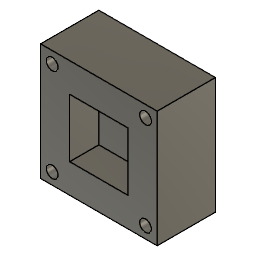
Milling (Autodesk Fusion 360 design; units mm, degrees)
part number: 2026-06-28-19-41-07-142
Autodesk Fusion 360 part; units mm, degrees
sketch "Sketch5" plane through (0, 0, 0) normal (0, 1, 0) x (1, 0, 0)
  line L0 (0, 0) -> (100, 0)
  line L1 (100, 0) -> (100, -100)
  line L2 (100, -100) -> (0, -100)
  line L3 (0, -100) -> (0, 0)
  line L4 (25, -75) -> (75, -75)
  line L5 (75, -75) -> (75, -25)
  line L6 (75, -25) -> (25, -25)
  line L7 (25, -25) -> (25, -75)
  circle A0 centre (10, -90) radius 5
  circle A1 centre (90, -90) radius 5
  circle A2 centre (90, -10) radius 5
  circle A3 centre (10, -10) radius 5
  dimension "d57" = 100
  dimension "d58" = 100
  dimension "d59" = 50
  dimension "d60" = 50
  dimension "d61" = 25
  dimension "d62" = 25
  dimension "d63" = 10
  dimension "d64" = 10
  dimension "d65" = 10
  dimension "d66" = 10
  constraint horizontal L0
  constraint vertical L1
  constraint horizontal L2
  constraint vertical L3
  constraint coincident L0.start L3.end
  constraint horizontal L4
  constraint vertical L5
  constraint horizontal L6
  constraint vertical L7
  measures "d57" distance of L1.end L2.end
  measures "d58" distance of L0.end L1.end
  measures "d59" distance of L4.start L4.end
  measures "d60" distance of L4.end L5.end
  measures "d61" distance of L1 L5
  measures "d62" distance of L2 L4
  measures "d63" diameter of A0
  measures "d64" diameter of A1
  measures "d65" diameter of A2
  measures "d66" diameter of A3
sketch "Sketch6" plane through (0, 0, 0) normal (0, 1, 0) x (1, 0, 0)
  line L0 (0, 0) -> (100, 0)
  line L1 (100, 0) -> (100, -100)
  line L2 (100, -100) -> (0, -100)
  line L3 (0, -100) -> (0, 0)
  line L4 (25, -75) -> (75, -75)
  line L5 (75, -75) -> (75, -25)
  line L6 (75, -25) -> (25, -25)
  line L7 (25, -25) -> (25, -75)
  circle A0 centre (10, -90) radius 5
  circle A1 centre (90, -90) radius 5
  circle A2 centre (90, -10) radius 5
  circle A3 centre (10, -10) radius 5
  line L8 (50, -100) -> (50, 0)
  line L9 (0, -50) -> (100, -50)
  dimension "d73" = 100
  dimension "d74" = 100
  dimension "d75" = 50
  dimension "d76" = 50
  dimension "d77" = 25
  dimension "d78" = 25
  dimension "d79" = 10
  dimension "d80" = 10
  dimension "d81" = 10
  dimension "d82" = 10
  constraint horizontal L0
  constraint vertical L1
  constraint horizontal L2
  constraint vertical L3
  constraint coincident L0.start L3.end
  constraint horizontal L4
  constraint vertical L5
  constraint horizontal L6
  constraint vertical L7
  constraint midpoint L2 L8.start
  constraint midpoint L0 L8.end
  constraint midpoint L3 L9.start
  constraint midpoint L1 L9.end
  measures "d73" distance of L0.start L2.end
  measures "d74" distance of L1.end L2.end
  measures "d75" distance of L4.start L4.end
  measures "d76" distance of L4.start L6.end
  measures "d77" distance of L1 L5
  measures "d78" distance of L2 L4
  measures "d79" diameter of A0
  measures "d80" diameter of A1
  measures "d81" diameter of A2
  measures "d82" diameter of A3
sketch "Sketch7" plane through (0, 0, 0) normal (0, 1, 0) x (1, 0, 0)
  line L0 (0, 0) -> (100, 0)
  line L1 (100, 0) -> (100, -100)
  line L2 (100, -100) -> (0, -100)
  line L3 (0, -100) -> (0, 0)
  line L4 (25, -75) -> (75, -75)
  line L5 (75, -75) -> (75, -25)
  line L6 (75, -25) -> (25, -25)
  line L7 (25, -25) -> (25, -75)
  circle A0 centre (10, -90) radius 5
  circle A1 centre (90, -90) radius 5
  circle A2 centre (90, -10) radius 5
  circle A3 centre (10, -10) radius 5
  line L8 (50, -100) -> (50, 0)
  line L9 (0, -50) -> (100, -50)
  dimension "d87" = 100
  dimension "d88" = 100
  dimension "d89" = 50
  dimension "d90" = 50
  dimension "d91" = 25
  dimension "d92" = 25
  dimension "d93" = 10
  dimension "d94" = 10
  dimension "d95" = 10
  dimension "d96" = 10
  constraint horizontal L0
  constraint vertical L1
  constraint horizontal L2
  constraint vertical L3
  constraint coincident L0.start L3.end
  constraint horizontal L4
  constraint vertical L5
  constraint horizontal L6
  constraint vertical L7
  constraint midpoint L2 L8.start
  constraint midpoint L0 L8.end
  constraint midpoint L3 L9.start
  constraint midpoint L1 L9.end
  measures "d87" distance of L0.end L1.end
  measures "d88" distance of L1.end L2.end
  measures "d89" distance of L4.start L4.end
  measures "d90" distance of L4.start L6.end
  measures "d91" distance of L1 L5
  measures "d92" distance of L2 L4
  measures "d93" diameter of A3
  measures "d94" diameter of A2
  measures "d95" diameter of A1
  measures "d96" diameter of A0
extrude "Extrude14" add sketch "Sketch7" along normal blind 50 contours L0 L3 L6 L7 L8 L9 | L0 L1 L5 L6 L8 L9 | L2 L3 L4 L7 L8 L9 | L6 L7 L8 L9 | L5 L6 L8 L9 | L4 L7 L8 L9 | L1 L2 L4 L5 L8 L9 | L4 L5 L8 L9 | A0 | A1 | A2 | A3
extrude "Extrude15" cut sketch "Sketch7" along normal blind 25 contours L6 L7 L8 L9 | L5 L6 L8 L9 | L4 L7 L8 L9 | L4 L5 L8 L9 | A0 | A1 | A2 | A3
